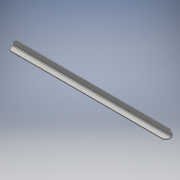
# Autodesk Inventor part: Part39
Saved by Autodesk Inventor 2016 (Build 200138000, 138)
## iProperties
Created: 2018-11-02
Part Number: Part39
Material: Generic
Document SubType Name: Sheet Metal
Designer: hovm
Density: 1 g/cm^3
Sheet Metal Rule: Default_mm
Appearance: Default
Author: hovm
Autodesk Inventor part; units mm, degrees
ref_plane "YZ Plane" through (0, 0, 0) normal (1, 0, 0) x (0, 1, 0)
ref_plane "XZ Plane" through (0, 0, 0) normal (0, 1, 0) x (-1, 0, 0)
ref_plane "XY Plane" through (0, 0, 0) normal (0, 0, 1) x (1, 0, 0)
sketch "Sketch1" plane through (0, 0, 0) normal (0, 0, 1) x (1, 0, 0)
  line L0 (-125, -5) -> (125, -5)
  line L1 (125, -5) -> (125, 5)
  line L2 (125, 5) -> (-125, 5)
  line L3 (-125, 5) -> (-125, -5)
  line L4 (-125, -5) -> (125, 5) construction
  line L5 (125, -5) -> (-125, 5) construction
  point P0 (0, 0)
  dimension "d0" = 250
  dimension "d1" = 10
  measures "d0" distance of L1.end L2.end
  measures "d1" distance of L0.end L1.end
extrude "Plate1" add sketch "Sketch1" along normal blind 1
sketch "Sketch2" plane through (-125, 4, 0) normal (0, 1, 0) x (-1, 0, 0)
  line L0 (-250, 0) -> (0, 0)
  line L1 (0, 0) -> (0, 10)
  line L2 (0, 10) -> (-250, 10)
  line L3 (-250, 10) -> (-250, 0)
  constraints: 6 end point, 1 horizontal, 1 perpendicular, 1 vertical
edge flange "Flange1" height 10 angle 90 thickness 1 bend radius 1 thickness toward (0, 1, 0) relief tear relief width 1 relief depth 0.5 edges at (0, 5, 1) wall of the first edge with corners at (125, 4, 0) (-125, 4, 0) (-125, 4, 10) (125, 4, 10)
bend "Bend1"
corner "Corner1"
chamfer "Corner Chamfer1" distance 4 angle 45 4 edges at (-125, 4.5, 10) (125, -5, 0.5) (125, 4.5, 10) (-125, -5, 0.5)
equation "\"d3\" = BendReliefWidth"
equation "\"d4\" = BendReliefDepth"
equation "\"d5\" = MinimumRemnant"
equation "\"d6\" = BendRadius"
equation "\"d9\" = BendRadius"
equation "\"d10\" = CornerReliefSize"
equation "\"d11\" = GapSize"
equation "\"d12\" = JacobiRadiusSize"
equation "\"BendRadius\" = Thickness"
equation "\"BendReliefWidth\" = Thickness"
equation "\"BendReliefDepth\" = 0.5 * Thickness"
equation "\"CornerReliefSize\" = 4 * Thickness"
equation "\"MinimumRemnant\" = 2 * Thickness"
equation "\"TransitionRadius\" = BendRadius"
equation "\"JacobiRadiusSize\" = BendRadius"
equation "\"GapSize\" = Thickness"
equation "\"d2\" = BendRadius"
equation "\"Thickness\" = 1"
body "Solid1"
